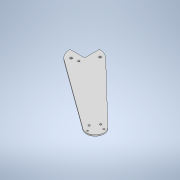
# Autodesk Inventor part: arm
Saved by Autodesk Inventor 2020 (Build 240168000, 168)
## iProperties
Created: 2019-06-21
Part Number: arm
Material: Generic
Document SubType Name: Modeling
Designer: Vivek Muskan
Density: 1 g/cm^3
Appearance: Default
Author: Vivek Muskan
Autodesk Inventor part; units mm, degrees
ref_plane "YZ Plane" through (0, 0, 0) normal (1, 0, 0) x (0, 1, 0)
ref_plane "XZ Plane" through (0, 0, 0) normal (0, 1, 0) x (-1, 0, 0)
ref_plane "XY Plane" through (0, 0, 0) normal (0, 0, 1) x (1, 0, 0)
sketch "Sketch1" plane through (0, 0, 0) normal (0, 1, 0) x (-1, 0, 0)
  line L0 (0, 0) -> (0, -25)
  line L1 (0, 0) -> (25, 0)
  line L2 (0, 0) -> (-107.2462, 89.9903)
  line L3 (0, 0) -> (140, 0) construction
  line L4 (-107.2462, 89.9903) -> (-102.7467, 95.3526)
  line L5 (-102.7467, 95.3526) -> (-110.9666, 84.0198)
  line L6 (-107.2462, 89.9903) -> (-114.9067, 96.4181)
  line L7 (-114.9067, 96.4181) -> (-120.6117, 88.2052)
  line L8 (-120.6117, 88.2052) -> (-109.2017, 104.6311)
  circle A0 centre (-109.2017, 104.6311) radius 1.5
  circle A1 centre (-102.7467, 95.3526) radius 1.5
  circle A2 centre (-110.9666, 84.0198) radius 1.5
  circle A3 centre (-120.6117, 88.2052) radius 1.5
  circle A4 centre (-111.0764, 93.2042) radius 15
  arc A5 (25, 0) -> (-19.1511, 16.0697) centre (0, 0) ccw
  arc A6 (-18.4671, 16.8513) -> (0, -25) centre (0, 0) ccw
  line L9 (-102.25, 105.3325) -> (14.7107, 20.2138)
  line L10 (-121.4878, 82.4058) -> (-17.3522, -17.9973)
  dimension "d0" = 25
  dimension "d1" = 25
  dimension "d2" = 140
  dimension "d3" = 140
  dimension "d4" = 7
  dimension "d5" = 14
  dimension "d6" = 10
  dimension "d7" = 10
  dimension "d8" = 20
  dimension "d9" = 3
  dimension "d10" = 3
  dimension "d11" = 3
  dimension "d12" = 3
  dimension "d13" = 30
  constraints: 22 end point, 8 point on circle, 7 centre point, 6 coincident, 4 tangent, 3 point on line, 2 horizontal, 1 equal length, 1 midpoint, 1 perpendicular, 1 vertical
  measures "d0" distance of L0.start L0.end
  measures "d1" distance of L0.start L1.end
  measures "d2" angle of L3 L2
  measures "d3" distance of L0.start L2.end
  measures "d4" distance of L2.end L4.end
  measures "d5" distance of L4.end L5.end
  measures "d6" distance of L2.end L6.end
  measures "d7" distance of L6.end L7.end
  measures "d8" distance of L7.end L8.end
  measures "d9" diameter of A0
  measures "d10" diameter of A1
  measures "d11" diameter of A2
  measures "d12" diameter of A3
  measures "d13" diameter of A4
extrude "Extrusion1" add sketch "Sketch1" along normal blind 2 contours L2 A5 L1 | L0 A6 L2 | A6 L10 A4 L2 | L2 A4 L9 A5 | L2 L4 A1 L5 | A4
sketch "Sketch2" plane through (0, 2, 0) normal (0, 1, 0) x (1, 0, 0)
  line L0 (0, 25) -> (0, 0) projected
  line L1 (0, 25) -> (0, 14)
  line L2 (0, 14) -> (12, 14)
  circle A0 centre (12, 14) radius 2
  line L3 (0, 25) -> (0, 0) projected
  line L4 (0, 0) -> (-10.922, 0)
  line L5 (0, 0) -> (-25, 0) projected
  line L6 (-10.922, 0) -> (-10.922, -12)
  circle A1 centre (-10.922, -12) radius 2
  dimension "d16" = 11
  dimension "d17" = 12
  dimension "d18" = 4
  dimension "d24" = 10.922
  dimension "d25" = 12
  dimension "d26" = 4
  constraints: 8 end point, 2 centre point, 2 coincident, 2 perpendicular, 2 point on line
  measures "d16" distance of L0.start L1.end
  measures "d17" distance of L1.end L2.end
  measures "d18" diameter of A0
  measures "d24" distance of L0.end L4.end
  measures "d25" distance of L4.end L6.end
  measures "d26" diameter of A1
extrude "Extrusion2" cut sketch "Sketch2" against normal blind 2 contours A0
extrude "Extrusion3" cut sketch "Sketch2" against normal blind 2 contours A1
sketch "Sketch3" plane through (0, 2, 0) normal (0, 1, 0) x (1, 0, 0)
  line L0 (0, 25) -> (0, 0) projected
  line L1 (0, 0) -> (0, -10)
  circle A0 centre (0, -10) radius 1.5
  dimension "d29" = 10
  dimension "d30" = 3
  constraints: 2 end point, 1 centre point, 1 coincident, 1 vertical
  measures "d29" distance of L0.end L1.end
  measures "d30" diameter of A0
extrude "Extrusion4" cut sketch "Sketch3" against normal blind 2
body "Solid1"
